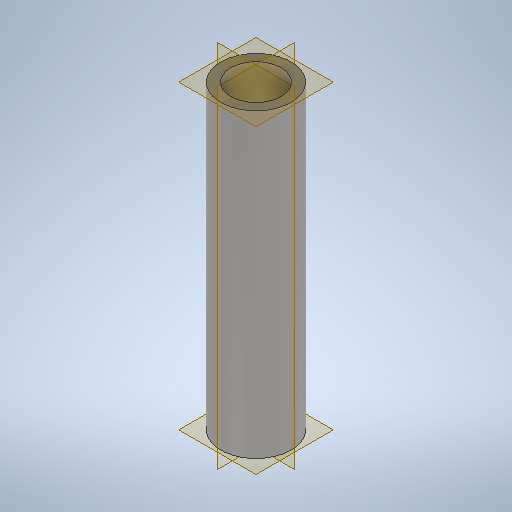
# Autodesk Inventor part: Z4
Saved by Autodesk Inventor 2025.2 (Build 292293000, 293)
## iProperties
Created: 2025-03-23
Part Number: Z4
Material: Steel, Alloy
Document SubType Name: Modeling
Designer: MSIGAMING
Mass: 48083.3 g
Surface Area: 4354.25 cm^2
Volume: 6220.35 cm^3
Density: 7.73 g/cm^3
Appearance: Semi-Polished
Author: MSIGAMING
Autodesk Inventor part; units mm, degrees
sketch "Sketch1" plane through (0, 0, 0) normal (0, 1, 0) x (-1, 0, 0)
  circle A0 centre (0, 0) radius 40
  circle A1 centre (0, 0) radius 70
  dimension "d0" = 80
  dimension "d1" = 140
  constraints: 2 centre point, 2 coincident
  measures "d0" diameter of A0
  measures "d1" diameter of A1
extrude "Extrusion1" add sketch "Sketch1" along normal blind 600
ref_plane "Work Plane1" through (0, 600, 0) normal (0, 1, 0) x (1, 0, 0)
sketch "Sketch3" plane through (0, 600, 0) normal (0, 1, 0) x (1, 0, 0)
  circle A0 centre (0, 0) radius 50
  circle A1 centre (0, 0) radius 40
  dimension "d5" = 100
  dimension "d6" = 80
  constraints: 2 centre point, 2 coincident
  measures "d5" diameter of A0
  measures "d6" diameter of A1
extrude "Extrusion2" cut sketch "Sketch3" against normal blind 180
body "Solid1"
